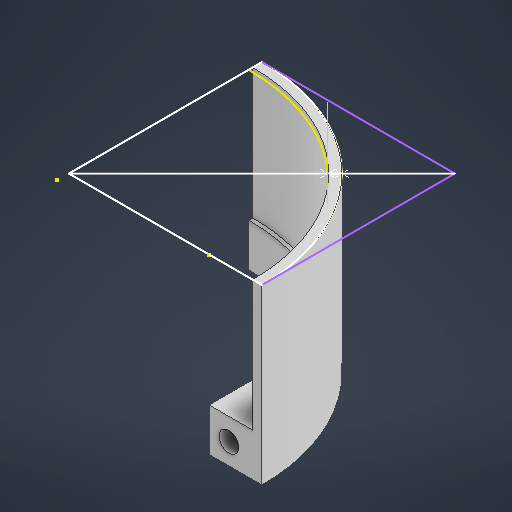
# Autodesk Inventor part: Conic_Cover
Saved by Autodesk Inventor 2026.2 (Build 302298000, 298)
## iProperties
Created: 2025-12-11
Part Number: Conic_Cover
Material: Generic
Document SubType Name: Modeling
Designer: Thoma
Density: 1 g/cm^3
Appearance: Default
Author: Thoma
Autodesk Inventor part; units mm, degrees
ref_plane "YZ Plane" through (0, 0, 0) normal (1, 0, 0) x (0, 1, 0)
ref_plane "XZ Plane" through (0, 0, 0) normal (0, 1, 0) x (-1, 0, 0)
ref_plane "XY Plane" through (0, 0, 0) normal (0, 0, 1) x (1, 0, 0)
sketch "Sketch1" plane through (0, 0, 0) normal (0, 1, 0) x (-1, 0, 0)
  line L0 (0, 0) -> (0, -36)
  line L1 (0, 0) -> (-12, 0)
  line L2 (0, 0) -> (42.5, 0)
  line L3 (42.5, 0) -> (42.5, -36)
  line L4 (0, -36) -> (42.5, -36)
  line L5 (42.5, -36) -> (42.5, -54.5)
  arc A0 (0, -36) -> (42.5, -54.5) centre (42.5, 3.5676) ccw
  line L6 (42.5, -54.5) -> (42.5, -58.5)
  circle A1 centre (42.5, 0) radius 58.5
  line L7 (-12, 0) -> (-16, 0)
  dimension "d0" = 36
  dimension "d1" = 42.5
  dimension "d2" = 18.5
  dimension "d3" = 4
  constraints: 16 end point, 4 point on circle, 4 vertical, 3 horizontal, 2 centre point, 2 perpendicular, 1 coincident, 1 line through centre
  measures "d0" distance of L0.start L0.end
  measures "d1" distance of L0.start L2.end
  measures "d2" distance of L3.end L5.end
  measures "d3" distance of L5.end L6.end
extrude "Extrusion1" add sketch "Sketch1" along normal blind 13 contours L0 A0 L6 A1 L7 L1
sketch "Sketch2" plane through (0, 13, 0) normal (0, 1, 0) x (1, 0, 0)
  arc A0 (0, 36) -> (-42.5, 54.5) centre (-42.5, -3.5676) ccw projected
  line L0 (0, 36) -> (2.1382, 37.8112)
  arc A1 (16, 0) -> (-42.5, 58.5) centre (-42.5, 0) ccw projected
  circle A2 centre (-42.5, 0) radius 58.5
  circle A3 centre (-42.5, 0) radius 55.6978
  line L1 (-42.5, 58.5) -> (-42.5, 54.5) projected
  line L2 (-42.5, 55.6978) -> (-42.5, 58.5)
  line L3 (0, 0) -> (16, 0) projected
  line L4 (13.1978, 0) -> (16, 0)
  dimension "d6" = 2.8022
  constraints: 6 end point, 4 point on circle, 2 centre point, 2 coincident, 2 collinear, 1 concentric, 1 line through centre
  measures "d6" distance of L0.start L0.end
extrude "Extrusion2" add sketch "Sketch2" along normal blind 39.5 contours A3 L1 A1 L0 | L0 A1 L3 A3
sketch "Sketch4" plane through (-42.5, 0, -58.5) normal (-1, 0, 0) x (0, 0, 1)
  line L0 (16, 92) -> (58.5, 92) projected
  line L1 (58.5, 105) -> (0, 105) projected
  line L2 (16, 92) -> (4, 92)
  line L3 (4, 92) -> (4, 105)
  line L4 (4, 105) -> (16, 105)
  line L5 (16, 105) -> (16, 92)
  circle A0 centre (10, 98.5) radius 3
  point P0 (58.5, 0)
  point P1 (0.0003, 105)
  dimension "d15" = 12
  dimension "d16" = 6
  constraints: 8 end point, 2 parallel, 1 centre point, 1 horizontal, 1 perpendicular, 1 point on line
  measures "d15" distance of L0.start L2.end
  measures "d16" diameter of A0
extrude "Extrusion4" cut sketch "Sketch4" against normal blind 5 contours A0
sketch "Sketch5" plane through (0, 0, 0) normal (0, 0, 1) x (1, 0, 0)
  line L0 (0, 0) -> (16, 0) projected
  line L1 (0, 13) -> (13.1978, 13) projected
  line L2 (0, 0) -> (12, 0)
  line L3 (12, 0) -> (12, 13)
  line L4 (12, 13) -> (0, 13)
  line L5 (0, 13) -> (0, 0)
  circle A0 centre (6, 6.3604) radius 3
  dimension "d19" = 6
  constraints: 8 end point, 2 parallel, 1 centre point, 1 horizontal, 1 perpendicular, 1 point on line
  measures "d19" diameter of A0
extrude "Extrusion5" cut sketch "Sketch5" against normal blind 5 contours A0
sketch "Sketch6" plane through (0, 52.5, 0) normal (0, 1, 0) x (1, 0, 0)
  arc A0 (16, 0) -> (-42.5, 58.5) centre (-42.5, 0) ccw projected
  line L0 (-42.5, 58.5) -> (-42.5, 0)
  line L1 (-42.5, 0) -> (16, 0)
  arc A1 (16, 0) -> (-42.5, 58.5) centre (-42.5, 0) ccw
  line L2 (-42.5, 0) -> (16, 0)
  line L3 (16, 0) -> (16, 58.5)
  line L4 (16, 58.5) -> (-42.5, 58.5)
  line L5 (-42.5, 58.5) -> (-42.5, 0)
  line L6 (-42.5, 0) -> (16, 58.5)
  arc A2 (0, 36) -> (-42.5, 54.5) centre (-42.5, -3.5676) ccw projected
  line L7 (-3.2626, 39.2374) -> (-1.1343, 41.3657)
  point P0 (0, 0)
  constraints: 16 end point, 4 point on circle, 2 parallel, 2 perpendicular, 2 point on line, 1 centre point, 1 collinear, 1 concentric, 1 horizontal, 1 vertical
ref_plane "Work Plane1" through (-3.2626, 52.5, -39.2374) normal (0.7071068, 0, -0.7071068) x (0, 1, 0)
body "Solid1"
